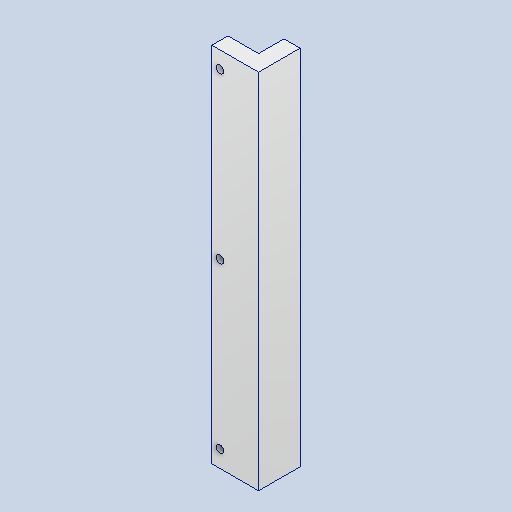
# Autodesk Inventor part: Guia lateral do top
Saved by Autodesk Inventor 2026 (Build 300175050, 175E)
## iProperties
Created: 2025-09-08
Part Number: Guia lateral do top
Material: Alumínio 6061
Document SubType Name: Modeling
Designer: Kedson Neves
Density: 2.7 g/cm^3
Appearance: Alumínio - Plano
Description: Guia lateral do top
Author: Kedson Neves
Autodesk Inventor part; units mm, degrees
ref_plane "YZ Plane" through (0, 0, 0) normal (1, 0, 0) x (0, 1, 0)
ref_plane "XZ Plane" through (0, 0, 0) normal (0, 1, 0) x (-1, 0, 0)
ref_plane "XY Plane" through (0, 0, 0) normal (0, 0, 1) x (1, 0, 0)
sketch "Esboço1" plane through (0, 0, 0) normal (0, 0, 1) x (1, 0, 0)
  line L0 (3.6169, 102.1463) -> (3.6169, -101.8537)
  line L1 (-13.8831, -106.8537) -> (-13.8831, 106.8093)
  line L2 (-13.8831, -106.8537) -> (-4.3831, -106.8537)
  line L3 (-13.8831, 106.8093) -> (-4.3831, 106.8093)
  circle A0 centre (-9.1331, -96.8537) radius 1.621
  circle A1 centre (-9.1331, -0.0222) radius 1.621
  circle A2 centre (-9.1331, 96.8093) radius 1.621
  line L4 (-13.8831, -106.8537) -> (13.6169, -106.8537)
  line L5 (13.6169, -106.8537) -> (13.6169, 106.8093)
  line L6 (13.6169, 106.8093) -> (-13.8831, 106.8093)
  line L7 (-13.8831, 106.8093) -> (-13.8831, -106.8537)
  point P0 (0, 0)
  point P1 (-13.8831, -10.6907)
  dimension "d0" = 0
  dimension "d1" = 10
  constraints: 16 end point, 3 centre point, 2 parallel, 1 horizontal, 1 perpendicular
  measures "d0" distance between parallel lines of L6 L3
  measures "d1" distance between parallel lines of L5 L0
extrude "Extrusão1" add sketch "Esboço1" along normal blind 9.5
sketch "Esboço2" plane through (0, 0, 0) normal (0, 0, -1) x (-1, 0, 0)
  line L0 (-13.6169, 106.8093) -> (13.8831, 106.8093) projected
  line L1 (13.8831, -106.8537) -> (-13.6169, -106.8537) projected
  line L2 (-13.6169, 106.8093) -> (-4.1169, 106.8093)
  line L3 (-4.1169, 106.8093) -> (-4.1169, -106.8537)
  line L4 (-4.1169, -106.8537) -> (-13.6169, -106.8537)
  line L5 (-13.6169, -106.8537) -> (-13.6169, 106.8093)
  point P0 (0, 0)
  dimension "d4" = 9.5
  constraints: 8 end point, 2 parallel, 1 horizontal, 1 perpendicular, 1 point on line
  measures "d4" distance between parallel lines of L5 L3
extrude "Extrusão2" add sketch "Esboço2" along normal blind 15
sketch "Esboço3" plane through (0, 0, 9.5) normal (0, 0, 1) x (1, 0, 0)
  circle A0 centre (-9.1331, -96.8537) radius 1.621 projected
  circle A1 centre (-9.1331, -0.0222) radius 1.621 projected
  circle A2 centre (-9.1331, 96.8093) radius 1.621 projected
  point P0 (0, 0)
  constraints: 3 coincident
hole "Furo1" at (-9.1331, -96.8537, 9.5) at (-9.1331, -0.0222, 9.5) at (-9.1331, 96.8093, 9.5) direction (0, 0, -1) diameter 4.5 end through all clearance for "Countersunk Flat Head Screw ISO 2009/7046" size "M4" standard "ISO"
